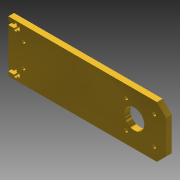
# Autodesk Inventor part: tiltColumnStepperSide02
Saved by Autodesk Inventor 2013 (Build 170138000, 138)
## iProperties
Created: 2014-06-14
Part Number: tiltColumnStepperSide02
Material: Gold
Document SubType Name: Modeling
Designer: Byron
Density: 19.3 g/cm^3
Mass: 1131.92 g
Surface Area: 227.905 cm^2
Volume: 58.6488 cm^3
Author: Byron
Autodesk Inventor part; units mm, degrees
note: some values were not read from the file. Chosen so that the rebuilt part matches the saved one: sketch regions of "Extrusion1".
ref_plane "YZ Plane" through (0, 0, 0) normal (1, 0, 0) x (0, 1, 0)
ref_plane "XZ Plane" through (0, 0, 0) normal (0, 1, 0) x (-1, 0, 0)
ref_plane "XY Plane" through (0, 0, 0) normal (0, 0, 1) x (1, 0, 0)
sketch "Sketch1" plane through (0, 0, 0) normal (0, 0, 1) x (1, 0, 0)
  circle A0 centre (-2.1414, -19.2098) radius 2 projected
  circle A1 centre (-31.9098, -10.5586) radius 2 projected
  circle A2 centre (6.5098, 10.5586) radius 2 projected
  circle A3 centre (-23.2586, 19.2098) radius 2 projected
  line L0 (-28.6845, 20.7851) -> (-21.6804, 24.6349) projected
  line L1 (-21.6804, 24.6349) -> (8.0851, 15.9845) projected
  line L2 (8.0851, 15.9845) -> (11.9349, 8.9804) projected
  line L3 (11.9349, 8.9804) -> (3.2845, -20.7851) projected
  line L4 (3.2845, -20.7851) -> (-3.7196, -24.6349) projected
  line L5 (-3.7196, -24.6349) -> (-33.4851, -15.9845) projected
  line L6 (-33.4851, -15.9845) -> (-37.3349, -8.9804) projected
  line L7 (-37.3349, -8.9804) -> (-28.6845, 20.7851) projected
  line L8 (9.5562, -25.8106) -> (19.9232, 9.8616)
  line L9 (19.9232, 9.8616) -> (13.1106, 22.2562)
  line L10 (13.1106, 22.2562) -> (-22.5616, 32.6232)
  line L11 (-22.5616, 32.6232) -> (-34.9562, 25.8106)
  line L12 (-34.9562, 25.8106) -> (-45.3232, -9.8616)
  line L13 (-45.3232, -9.8616) -> (-38.5106, -22.2562)
  line L14 (-38.5106, -22.2562) -> (-2.8384, -32.6232)
  line L15 (-2.8384, -32.6232) -> (9.5562, -25.8106)
  line L16 (-38.5106, -22.2562) -> (-165.5106, -22.2562)
  line L17 (-165.5106, -22.2562) -> (-165.5106, 34.8938)
  line L18 (-165.5106, 34.8938) -> (-38.5106, 34.8938)
  line L19 (-38.5106, 34.8938) -> (-38.5106, -22.2562)
  circle A4 centre (-12.7, 0) radius 11 projected
  point P0 (0, 0)
  dimension "d0" = 127
  dimension "d1" = 57.15
  dimension "d2" = 57.15
  constraints: 24 end point, 2 parallel, 1 horizontal, 1 perpendicular, 7 other
  measures "d0" distance of L17.end L18.end
  measures "d1" distance between parallel lines of L10 L14
  measures "d2" distance of L16.end L17.end
extrude "Extrusion1" add sketch "Sketch1" along normal blind 6.35 contours L0 L1 L2 L3 L4 L5 L6 L7 | L15 L14 L19 L12 L11 L10 L9 L8 | L16 L17 L18 L19 L12 L13 | L13 L12 L19
sketch "Sketch2" plane through (0, 0, 0) normal (0, 0, -1) x (-1, 0, 0)
  line L0 (136.7986, -16.3493) -> (136.7986, -9.9993) projected
  line L1 (133.0902, -9.9993) -> (133.0902, -16.3493) projected
  line L2 (136.7986, 9.0507) -> (136.7986, 15.4007) projected
  line L3 (133.0902, 15.4007) -> (133.0902, 9.0507) projected
  line L4 (126.7402, -12.7) -> (130.4486, -12.7) construction
  line L5 (126.7402, 12.7) -> (130.4486, 12.7) construction
  circle A0 centre (128.5944, -12.7) radius 1.8542
  circle A1 centre (128.5944, 12.7) radius 1.8542
  dimension "d5" = 3.7084
  dimension "d6" = 3.7084
  constraints: 4 end point, 2 centre point
  measures "d5" diameter of A0
  measures "d6" diameter of A1
extrude "Extrusion2" cut sketch "Sketch2" against normal through all
sketch "Sketch3" plane through (0, 0, 0) normal (0, 0, -1) x (-1, 0, 0)
  line L0 (165.5106, 34.8938) -> (165.5106, -22.2562) projected
  line L1 (153.1125, 15.7309) -> (159.2102, 17.5031) projected
  line L2 (170.3558, -20.8481) -> (159.2102, 17.5031) projected
  line L3 (2.8384, -32.6232) -> (155.6197, 11.7778) projected
  line L4 (-9.5562, -25.8106) -> (2.8384, -32.6232) projected
  line L5 (-19.9232, 9.8616) -> (-9.5562, -25.8106) projected
  line L6 (-13.1106, 22.2562) -> (-19.9232, 9.8616) projected
  line L7 (154.986, 71.1081) -> (-13.1106, 22.2562) projected
  line L8 (145.7706, 63.7481) -> (155.0405, 31.851) projected
  line L9 (145.7706, 63.7481) -> (139.6729, 61.976) projected
  line L10 (139.6729, 61.976) -> (139.0916, 63.9761) projected
  line L11 (139.0916, 63.9761) -> (136.4086, 63.1964) projected
  line L12 (136.4086, 63.1964) -> (136.9899, 61.1963) projected
  line L13 (136.9899, 61.1963) -> (133.5752, 60.2039) projected
  line L14 (133.5752, 60.2039) -> (134.6101, 56.6429) projected
  line L15 (134.6101, 56.6429) -> (138.0248, 57.6352) projected
  line L16 (138.0248, 57.6352) -> (138.606, 55.6352) projected
  line L17 (138.606, 55.6352) -> (141.289, 56.4149) projected
  line L18 (141.289, 56.4149) -> (140.7078, 58.415) projected
  line L19 (140.7078, 58.415) -> (146.8055, 60.1871) projected
  line L20 (158.1753, 21.0641) -> (146.8055, 60.1871) projected
  line L21 (158.1753, 21.0641) -> (152.0776, 19.292) projected
  line L22 (152.0776, 19.292) -> (151.4964, 21.2921) projected
  line L23 (151.4964, 21.2921) -> (148.8134, 20.5123) projected
  line L24 (148.8134, 20.5123) -> (149.3946, 18.5123) projected
  line L25 (149.3946, 18.5123) -> (145.9799, 17.5199) projected
  line L26 (145.9799, 17.5199) -> (147.0148, 13.9588) projected
  line L27 (147.0148, 13.9588) -> (150.4295, 14.9512) projected
  line L28 (150.4295, 14.9512) -> (151.0108, 12.9512) projected
  line L29 (151.0108, 12.9512) -> (153.6938, 13.7309) projected
  line L30 (153.6938, 13.7309) -> (153.1125, 15.7309) projected
  circle A0 centre (132.6412, 48.0825) radius 1.8542 projected
  circle A1 centre (139.7296, 23.6916) radius 1.8542 projected
  circle A2 centre (2.1414, -19.2098) radius 2 projected
  circle A3 centre (31.9098, -10.5586) radius 2 projected
  circle A4 centre (-6.5098, 10.5586) radius 2 projected
  circle A5 centre (23.2586, 19.2098) radius 2 projected
  circle A6 centre (12.7, 0) radius 11 projected
  point P0 (165.5106, -22.2562)
  constraints: 3 other
extrude "Extrusion3" [suppressed]
equation "\"d2\" = d1"
body "Solid1"
